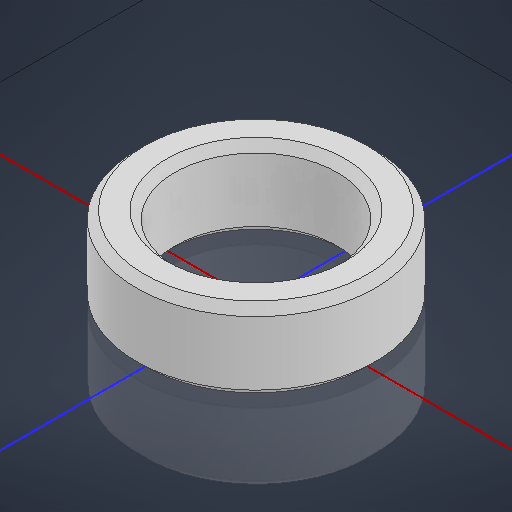
# Autodesk Inventor part: Case Bottom Ring
Saved by Autodesk Inventor 2026 (Build 300175000, 175)
## iProperties
Created: 2025-06-07
Part Number: Case Bottom Ring
Material: Generic
Document SubType Name: Modeling
Designer: ckyiu
Density: 1 g/cm^3
Appearance: Default
Author: ckyiu
Autodesk Inventor part; units mm, degrees
ref_plane "YZ Plane" through (0, 0, 0) normal (1, 0, 0) x (0, 1, 0)
ref_plane "XZ Plane" through (0, 0, 0) normal (0, 1, 0) x (-1, 0, 0)
ref_plane "XY Plane" through (0, 0, 0) normal (0, 0, 1) x (1, 0, 0)
sketch "Sketch1" plane through (0, 0, 0) normal (0, 1, 0) x (-1, 0, 0)
  circle A0 centre (0, 0) radius 7.5
  dimension "d0" = 15
  constraints: 1 centre point, 1 coincident
  measures "d0" diameter of A0
extrude "Extrusion1" add sketch "Sketch1" along normal blind 5
sketch "Sketch2" plane through (0, 5, 0) normal (0, 1, 0) x (1, 0, 0)
  point P0 (0, 0)
  point P1 (0, 0)
  constraints: 1 coincident
hole "Hole1" at (0, 5, 0) direction (0, -1, 0) diameter 10.2 end through all
chamfer "Chamfer1" distance 0.5 angle 45 4 edges at (7.5, 5, 0) (0, 5, -5.1) (0, 0, -5.1) (7.5, 0, 0)
body "Solid1"
